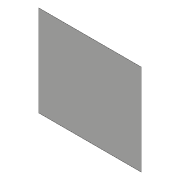
# Autodesk Inventor part: plinthScreen
Saved by Autodesk Inventor 2017 (Build 210142000, 142)
## iProperties
Created: 2016-11-30
Part Number: plinthScreen
Material: Generic
Document SubType Name: Modeling
Designer: krosie
Density: 1 g/cm^3
Appearance: Default
Author: krosie
Autodesk Inventor part; units mm, degrees
ref_plane "YZ Plane" through (0, 0, 0) normal (1, 0, 0) x (0, 1, 0)
ref_plane "XZ Plane" through (0, 0, 0) normal (0, 1, 0) x (-1, 0, 0)
ref_plane "XY Plane" through (0, 0, 0) normal (0, 0, 1) x (1, 0, 0)
sketch "Sketch3" plane through (0, 0, 0) normal (0, 1, 0) x (-1, 0, 0)
  line L0 (-450, 400) -> (450, 400)
  line L1 (450, 400) -> (450, -400)
  line L2 (450, -400) -> (-450, -400)
  line L3 (-450, -400) -> (-450, 400)
  line L4 (-450, 400) -> (450, -400) construction
  line L5 (450, 400) -> (-450, -400) construction
  point P0 (0, 0)
  dimension "d8" = 900
  dimension "d9" = 800
  constraints: 12 end point, 2 midpoint, 2 parallel, 1 horizontal, 1 perpendicular
  measures "d8" distance of L1.end L2.end
  measures "d9" distance of L0.end L1.end
extrude "Extrusion1" add sketch "Sketch3" along normal blind 0.71
body "Solid2"
